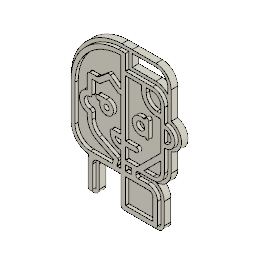
femIT_keychain (Autodesk Fusion 360 design; units mm, degrees)
Autodesk Fusion 360 part; units mm, degrees
sketch "MAIN" plane through (0, 0, 0) normal (0, 1, 0) x (1, 0, 0)
  line L0 (17.9916, -4.7059) -> (17.9916, -8.3513)
  line L1 (-9.0064, 3.7559) -> (-9.0064, -7.1582)
  line L2 (9.3752, 7.8431) -> (9.3752, 7.3129)
  arc A0 (12.3525, -3.3087) -> (13.2635, -3.4243) centre (12.8027, -3.4084) cw
  line L3 (3.167, 0.9058) -> (4.7357, 0.9058)
  line L4 (0.5265, -7.4454) -> (-1.9697, -7.4454)
  circle A1 centre (0.5265, -5.3563) radius 0.773
  arc A2 (-1.7946, -12.1762) -> (-2.4001, -11.97) centre (-2.4001, -12.9622) ccw
  arc A3 (18.0688, -9.5664) -> (17.9916, -9.6548) centre (18.0808, -9.6548) ccw
  spline S0 degree 3 poles (6.3043, 5.5675) (6.2676, 5.5675) (6.238, 5.5379) (6.238, 5.5012) knots 0 0 0 0 1 1 1 1
  spline S1 degree 3 poles (15.8928, 11.4887) (15.8928, 9.8013) (14.52, 8.4286) (12.8328, 8.4286) knots 0 0 0 0 1 1 1 1
  line L5 (6.3043, 6.7384) -> (7.8729, 6.7384)
  line L6 (4.5195, -12.2526) -> (1.6695, -14.3514)
  arc A4 (13.352, 9.8755) -> (14.4567, 11.0258) centre (13.352, 10.9811) ccw
  arc A5 (4.7303, -21.1201) -> (4.7964, -21.0671) centre (4.7314, -21.0537) ccw
  line L7 (4.7356, -12.2397) -> (4.5589, -12.2397)
  line L8 (2.5786, 7.2131) -> (2.2251, 8.3619)
  line L9 (-2.3821, 4.7038) -> (2.5445, 7.1341)
  arc A6 (12.1671, -8.257) -> (11.649, -8.0278) centre (11.8064, -8.3722) ccw
  arc A7 (-5.15, 9.5279) -> (-4.9416, 10.21) centre (-5.2035, 9.9172) ccw
  line L10 (6.238, -17.7188) -> (6.238, -22.2923)
  line L11 (7.9394, 6.8047) -> (7.9394, 8.3734)
  line L12 (9.6625, 5.5675) -> (6.3043, 5.5675)
  line L13 (-10.1773, -7.4786) -> (-10.1773, 3.865)
  line L14 (6.238, -22.2923) -> (4.1436, -22.2923)
  arc A8 (-5.2726, -7.0697) -> (-5.3234, -7.0131) centre (-5.3389, -7.0782) ccw
  arc A9 (-5.3234, -7.0131) -> (-5.3234, -1.1028) centre (-4.619, -4.058) cw
  arc A10 (4.7357, 2.1526) -> (3.1081, 0.9938) centre (4.7357, 0.4303) ccw
  arc A11 (-4.5662, -11.97) -> (-5.2726, -11.253) centre (-4.5556, -11.253) cw
  line L15 (17.9916, -9.6548) -> (17.9916, -14.0624)
  line L16 (4.7964, -21.0671) -> (4.8019, -12.306)
  arc A12 (-1.9697, -7.4454) -> (-1.9697, -6.0092) centre (-1.9697, -6.7273) cw
  arc A13 (18.0579, -4.6396) -> (17.9916, -4.7059) centre (18.0579, -4.7059) ccw
  line L17 (4.8019, 9.942) -> (4.8019, 17.8735)
  arc A14 (-5.2726, 0) -> (-2.3821, 4.7038) centre (0, 0) cw
  arc A15 (12.0111, -3.4605) -> (12.3525, -3.3087) centre (12.1257, -3.2584) ccw
  line L18 (-5.2726, -1.0382) -> (-5.2726, 0)
  arc A16 (9.4415, 0.5523) -> (9.4194, 1.9884) centre (9.4194, 1.2702) ccw
  arc A17 (13.2635, -8.0861) -> (12.1671, -8.257) centre (12.702, -8.0861) cw
  arc A18 (4.5589, -12.2397) -> (4.5195, -12.2526) centre (4.5587, -12.3059) ccw
  spline S2 degree 3 poles (6.3043, 17.4095) (6.2676, 17.4095) (6.238, 17.3799) (6.238, 17.3432) knots 0 0 0 0 1 1 1 1
  arc A19 (6.3043, -17.6525) -> (6.238, -17.7188) centre (6.3043, -17.7188) ccw
  line L19 (6.3043, 9.8755) -> (13.352, 9.8755)
  arc A20 (2.2251, 8.3619) -> (2.1616, 8.4085) centre (2.162, 8.3425) ccw
  arc A21 (17.9916, -8.3513) -> (18.0579, -8.4175) centre (18.0579, -8.3513) ccw
  spline S3 degree 3 poles (-10.1773, 3.865) (-10.1256, 6.7548) (-8.012, 9.1345) (-5.15, 9.5279) knots 0 0 0 0 1 1 1 1
  arc A22 (11.649, -8.0278) -> (12.0111, -3.4605) centre (10.7656, -5.6598) cw
  arc A23 (6.238, 2.0547) -> (6.3043, 1.9884) centre (6.3043, 2.0547) ccw
  line L20 (-5.2726, -11.253) -> (-5.2726, -7.0697)
  spline S4 degree 3 poles (9.9607, 8.4286) (9.6378, 8.4286) (9.3752, 8.1661) (9.3752, 7.8431) knots 0 0 0 0 1 1 1 1
  line L21 (0.7791, -14.3317) -> (-1.7946, -12.1762)
  line L22 (15.6827, -10.4943) -> (16.7544, -10.4943)
  arc A24 (-4.3557, 8.4085) -> (-9.0064, 3.7559) centre (-4.3557, 3.7579) ccw
  line L23 (5.7851, 18.8566) -> (14.9096, 18.8566)
  arc A25 (-1.5388, -6.0092) -> (-1.4815, -5.9331) centre (-1.5388, -5.9495) ccw
  arc A26 (-5.3234, -1.1028) -> (-5.2726, -1.0382) centre (-5.3388, -1.0385) ccw
  line L24 (6.238, 17.3432) -> (6.238, 9.942)
  line L25 (-1.9697, -6.0092) -> (-1.5388, -6.0092)
  line L26 (-2.4001, -11.97) -> (-4.5662, -11.97)
  arc A27 (-9.0064, -7.1582) -> (4.7303, -21.1201) centre (4.9573, -7.1582) ccw
  arc A28 (2.5445, 7.1341) -> (2.5786, 7.2131) centre (2.5152, 7.1936) ccw
  line L27 (2.1616, 8.4085) -> (-4.3557, 8.4085)
  circle A29 centre (4.7357, 2.0863) radius 0.0663
  spline S5 degree 3 poles (9.7092, 5.5482) (9.6969, 5.5605) (9.6799, 5.5675) (9.6625, 5.5675) knots 0 0 0 0 1 1 1 1
  line L28 (15.8928, 17.8735) -> (15.8928, 11.4887)
  arc A30 (1.6695, -14.3514) -> (0.7791, -14.3317) centre (1.2366, -13.7855) cw
  arc A31 (18.0579, -8.4175) -> (18.0579, -4.6396) centre (18.0579, -6.5286) ccw
  arc A32 (4.8019, -12.306) -> (4.7356, -12.2397) centre (4.7356, -12.306) ccw
  line L29 (6.238, 8.3734) -> (6.238, 6.8047)
  arc A33 (-1.4815, -5.9331) -> (0.5265, -7.4454) centre (0.5265, -5.3563) cw
  line L30 (13.2635, -3.4243) -> (13.2635, -8.0861)
  spline S6 degree 3 poles (-3.8353, 0.0055) (-3.8354, 0.0037) (-3.8365, 0.002) (-3.8365, 0) knots 0 0 0 0 1 1 1 1
  spline S7 degree 3 poles (7.9394, 8.3734) (7.9394, 8.41) (7.9095, 8.4396) (7.8729, 8.4396) knots 0 0 0 0 1 1 1 1
  line L31 (16.8209, 0.6188) -> (16.8209, 3.4024)
  spline S8 degree 3 poles (7.8729, 6.7384) (7.9095, 6.7384) (7.9394, 6.7681) (7.9394, 6.8047) knots 0 0 0 0 1 1 1 1
  arc A34 (3.1081, 0.9938) -> (3.1707, 0.9058) centre (3.1707, 0.9721) ccw
  line L32 (7.8729, 8.4396) -> (6.3043, 8.4396)
  spline S9 degree 3 poles (14.9096, 18.8566) (15.4516, 18.8566) (15.8928, 18.4155) (15.8928, 17.8735) knots 0 0 0 0 1 1 1 1
  line L33 (4.8019, 3.7021) -> (4.8019, 8.3513)
  arc A35 (14.3904, -17.6525) -> (17.9916, -14.0624) centre (14.3904, -14.0513) ccw
  spline S10 degree 3 poles (4.7357, 9.8755) (4.7723, 9.8755) (4.8019, 9.9052) (4.8019, 9.942) knots 0 0 0 0 1 1 1 1
  spline S11 degree 3 poles (6.238, 9.942) (6.238, 9.9052) (6.2676, 9.8755) (6.3043, 9.8755) knots 0 0 0 0 1 1 1 1
  arc A36 (4.7357, 0.9058) -> (4.8019, 0.9721) centre (4.7357, 0.9721) ccw
  arc A37 (16.7544, -10.4943) -> (16.8209, -10.428) centre (16.7544, -10.4278) ccw
  line L34 (14.6553, 5.5675) -> (11.8716, 5.5675)
  line L35 (-2.047, 9.8755) -> (4.7357, 9.8755)
  arc A38 (17.9916, 3.1373) -> (14.3794, 6.7274) centre (14.3794, 3.1151) ccw
  arc A39 (16.7074, 0.5718) -> (16.8209, 0.6188) centre (16.7544, 0.6188) ccw
  arc A40 (-3.6596, 11.4887) -> (-2.047, 9.8755) centre (-2.0464, 11.4887) ccw
  line L36 (11.8248, 5.4543) -> (16.7074, 0.5718)
  arc A41 (5.7851, 18.8566) -> (4.8019, 17.8735) centre (5.7851, 17.8735) ccw
  arc A42 (-3.6596, 18.1167) -> (-5.0959, 18.1167) centre (-4.3777, 18.1167) ccw
  arc A43 (11.8716, 5.5675) -> (11.8248, 5.4543) centre (11.8717, 5.5012) ccw
  arc A44 (-10.1773, -7.4786) -> (4.1436, -22.2923) centre (4.6449, -7.4786) ccw
  spline S12 degree 3 poles (14.4567, 17.3432) (14.4567, 17.3799) (14.4271, 17.4095) (14.3904, 17.4095) knots 0 0 0 0 1 1 1 1
  spline S13 degree 3 poles (-3.8365, 0.011) (-3.8365, 0.0092) (-3.8354, 0.0074) (-3.8353, 0.0055) knots 0 0 0 0 1 1 1 1
  line L37 (4.7356, -0.5302) -> (2.206, -0.5302)
  spline S14 degree 3 poles (6.3043, 8.4396) (6.2676, 8.4396) (6.238, 8.41) (6.238, 8.3734) knots 0 0 0 0 1 1 1 1
  arc A45 (2.206, -0.5302) -> (1.5982, 0.0773) centre (2.206, 0.0775) cw
  line L38 (14.4567, 11.0258) -> (14.4567, 17.3432)
  line L39 (12.8328, 8.4286) -> (9.9607, 8.4286)
  arc A46 (15.6827, -10.4943) -> (11.0543, -15.1118) centre (15.6718, -15.1118) ccw
  arc A47 (-5.0959, 10.5483) -> (-4.9416, 10.21) centre (-4.633, 10.5551) ccw
  line L40 (14.3904, 17.4095) -> (6.3043, 17.4095)
  line L41 (1.5982, 0.0773) -> (1.5982, 0.4419)
  line L42 (4.8019, 0.9721) -> (4.8019, 2.0863)
  arc A48 (6.3043, 0.5523) -> (6.238, 0.4861) centre (6.3043, 0.4861) ccw
  arc A49 (4.6891, 3.5983) -> (4.8019, 3.7021) centre (4.6977, 3.7021) ccw
  arc A50 (10.9881, -16.4814) -> (11.0543, -16.4151) centre (10.9881, -16.4151) ccw
  arc A51 (1.5982, 0.4419) -> (4.6891, 3.5983) centre (4.7553, 0.4419) cw
  line L43 (-5.0959, 10.5483) -> (-5.0959, 18.1167)
  arc A52 (16.8209, 3.4024) -> (14.6553, 5.5675) centre (14.6553, 3.402) ccw
  arc A53 (4.8019, 8.3513) -> (4.7356, 8.4175) centre (4.7356, 8.3513) ccw
  arc A54 (18.0025, -3.3804) -> (18.0688, -3.4465) centre (18.0688, -3.3803) ccw
  line L44 (-3.6596, 18.1167) -> (-3.6596, 11.4887)
  arc A55 (18.0688, -9.5664) -> (18.0688, -3.4465) centre (18.0688, -6.5065) ccw
  line L45 (9.9607, 6.7274) -> (14.3794, 6.7274)
  circle A56 centre (10.7656, -5.6598) radius 1.2113
  spline S15 degree 3 poles (6.238, 6.8047) (6.238, 6.7681) (6.2676, 6.7384) (6.3043, 6.7384) knots 0 0 0 0 1 1 1 1
  line L46 (4.7356, 8.4175) -> (3.6974, 8.4175)
  arc A57 (6.238, -16.4151) -> (6.3043, -16.4814) centre (6.3043, -16.4151) ccw
  arc A58 (-1.6686, 3.4447) -> (-3.8365, 0) centre (-0.0158, 0) ccw
  arc A59 (4.1181, 6.7692) -> (3.8886, 6.2231) centre (3.6781, 6.6329) cw
  line L47 (-3.8365, 0) -> (-3.8365, -1.705)
  line L48 (3.6341, 8.3317) -> (4.1181, 6.7692)
  line L49 (3.8886, 6.2231) -> (-1.6686, 3.4447)
  arc A60 (3.6974, 8.4175) -> (3.6341, 8.3317) centre (3.6974, 8.3513) ccw
  arc A61 (-4.5807, -5.6331) -> (-3.8365, -6.3629) centre (-4.5607, -6.357) cw
  line L50 (6.3043, -16.4814) -> (10.9881, -16.4814)
  line L51 (-3.7703, -10.5385) -> (-1.5188, -10.5385)
  arc A62 (16.8209, -11.9967) -> (16.7544, -11.9304) centre (16.7544, -11.9968) ccw
  arc A63 (14.3904, -16.4814) -> (16.8209, -14.0734) centre (14.3904, -14.0509) ccw
  line L52 (17.9916, 3.1373) -> (18.0025, -3.3804)
  line L53 (16.8013, -1.5438) -> (9.7092, 5.5482)
  arc A64 (-4.6209, -2.4303) -> (-4.5807, -5.6331) centre (-4.6209, -4.0319) ccw
  arc A65 (1.2243, -12.8428) -> (1.3064, -12.8454) centre (1.267, -12.792) ccw
  line L54 (11.0543, -16.4151) -> (11.0543, -15.1118)
  line L55 (16.8209, -14.0734) -> (16.8209, -11.9967)
  arc A66 (-3.8365, -1.705) -> (-4.6209, -2.4303) centre (-4.6209, -1.6435) cw
  line L56 (12.5567, -16.4814) -> (14.3904, -16.4814)
  line L57 (-3.8365, -6.3629) -> (-3.8365, -10.4722)
  arc A67 (4.8019, -0.5965) -> (4.7356, -0.5302) centre (4.7356, -0.5965) ccw
  line L58 (6.238, 0.4861) -> (6.238, -16.4151)
  line L59 (4.0725, -10.8036) -> (4.7356, -10.8036)
  arc A68 (4.7356, -10.8036) -> (4.8019, -10.7373) centre (4.7356, -10.7373) ccw
  line L60 (1.3064, -12.8454) -> (4.0725, -10.8036)
  arc A69 (-3.8365, -10.4722) -> (-3.7703, -10.5385) centre (-3.7703, -10.4722) ccw
  line L61 (4.8019, -10.7373) -> (4.8019, -0.5965)
  line L62 (-1.5188, -10.5385) -> (1.2243, -12.8428)
  line L63 (9.4415, 0.5523) -> (6.3043, 0.5523)
  arc A70 (12.4904, -16.4151) -> (12.5567, -16.4814) centre (12.5567, -16.4151) ccw
  spline S16 degree 3 poles (9.3752, 7.3129) (9.3752, 6.9901) (9.6378, 6.7274) (9.9607, 6.7274) knots 0 0 0 0 1 1 1 1
  line L64 (12.4904, -15.1118) -> (12.4904, -16.4151)
  line L65 (6.238, 5.5012) -> (6.238, 2.0547)
  line L66 (6.3043, 1.9884) -> (9.4194, 1.9884)
  line L67 (16.8209, -10.428) -> (16.8209, -1.5907)
  arc A71 (15.6718, -11.9304) -> (12.4904, -15.1118) centre (15.6718, -15.1118) ccw
  line L68 (16.7544, -11.9304) -> (15.6718, -11.9304)
  line L69 (14.3904, -17.6525) -> (6.3043, -17.6525)
  spline S17 degree 3 poles (16.8209, -1.5907) (16.8209, -1.573) (16.8137, -1.5563) (16.8013, -1.5438) knots 0 0 0 0 1 1 1 1
  line L70 (7.238, -23.2923) -> (4.1269, -23.2923)
  arc A72 (-11.1773, -7.4786) -> (4.1269, -23.2923) centre (4.6449, -7.4786) ccw
  line L71 (-11.1773, -7.4786) -> (-11.1773, 3.874)
  spline S18 degree 3 poles (-11.1773, 3.874) (-11.1773, 3.877) (-11.1772, 3.88) (-11.1772, 3.8829) (-11.1218, 6.9765) (-9.0162, 9.6026) (-6.083, 10.3615) knots -0.001032 -0.001032 -0.001032 -0.001032 0 0 0 0.918689 0.918689 0.918689 0.918689
  arc A73 (-6.0959, 10.5429) -> (-6.083, 10.3615) centre (-4.633, 10.5551) ccw
  line L72 (-6.0959, 10.5429) -> (-6.0959, 18.1167)
  arc A74 (-2.6596, 18.1167) -> (-6.0959, 18.1167) centre (-4.3777, 18.1167) ccw
  line L73 (-2.6596, 18.1167) -> (-2.6596, 11.4887)
  arc A75 (-2.6596, 11.4887) -> (-2.0462, 10.8755) centre (-2.0464, 11.4887) ccw
  line L74 (-2.0462, 10.8755) -> (3.8019, 10.8755)
  line L75 (3.8019, 10.8755) -> (3.8019, 17.8735)
  arc A76 (5.7851, 19.8566) -> (3.8019, 17.8735) centre (5.7851, 17.8735) ccw
  line L76 (5.7851, 19.8566) -> (14.9096, 19.8566)
  spline S19 degree 3 poles (14.9096, 19.8566) (15.8842, 19.8566) (16.7097, 19.1405) (16.866, 18.1986) (16.8837, 18.0923) (16.8928, 17.9834) (16.8928, 17.8735) knots 0 0 0 0 0.898599 0.898599 0.898599 1 1 1 1
  line L77 (16.8928, 17.8735) -> (16.8928, 11.4887)
  spline S20 degree 3 poles (16.8928, 11.4887) (16.8928, 9.7969) (15.8471, 8.3329) (14.3617, 7.7274) knots 0 0 0 0 0.758742 0.758742 0.758742 0.758742
  line L78 (14.3617, 7.7274) -> (14.3794, 7.7274)
  arc A77 (18.9916, 3.141) -> (14.3794, 7.7274) centre (14.3794, 3.1151) ccw
  line L79 (18.9916, 3.141) -> (19.0011, -2.5551)
  arc A78 (18.9916, -10.4601) -> (19.0011, -2.5551) centre (18.0688, -6.5065) ccw
  line L80 (18.9916, -10.4601) -> (18.9916, -14.0638)
  arc A79 (14.3904, -18.6525) -> (18.9916, -14.0638) centre (14.3904, -14.0513) ccw
  line L81 (14.3904, -18.6525) -> (7.238, -18.6525)
  line L82 (7.238, -18.6525) -> (7.238, -23.2923)
  line L83 (7.238, -23.2923) -> (21.9939, -23.2923)
  line L84 (18.9916, -14.0638) -> (18.9916, -25.254)
  arc A80 (14.3904, -23.2923) -> (18.9916, -18.6911) centre (14.3904, -18.6911) ccw
  arc A81 (14.3904, -22.2923) -> (17.9916, -18.6911) centre (14.3904, -18.6911) ccw
  line L85 (14.3904, -22.2923) -> (7.238, -22.2923)
  line L86 (17.9916, -18.6911) -> (17.9916, -16.9153)
  line L87 (5.7851, 19.8566) -> (-4.3777, 19.8348)
  dimension "d6" = 1
  dimension "d7" = -1
  constraint horizontal L83
  constraint perpendicular L82 L83
  constraint vertical L84
  constraint tangent L83 A80
  constraint tangent L84 A80
  constraint equal A79 A80
  constraint coincident L83 A80.start
  constraint coincident L84 A80.end
  constraint coincident L82 L85.end
  constraint tangent A81 L85
  constraint perpendicular L82 L85
  constraint coincident A79 L86.end
  constraint tangent A81 L86
  constraint vertical L86
  constraint midpoint A74 L87.end
extrude "Extrude1" add sketch "MAIN" along normal blind 2 contours L0 A13 A21 A31 | L1 A2 L6 A5 L7 L8 L9 A8 A9 A11 L16 A14 L18 A18 A20 L20 L21 A24 A26 L26 A27 A28 L27 A30 A32 | L2 A3 S1 A7 L10 L13 L14 L15 L17 A19 S3 S4 L23 L28 S9 A35 S10 L35 A38 A40 A41 A42 A44 L39 A47 L43 A54 L44 A55 L45 L52 S16 L69 | A0 A6 A15 A17 A22 L30 | L3 A10 A29 A34 A36 L42 | L4 A12 A25 L25 A33 | A1 | S0 L12 A16 A23 L22 S5 A37 A46 A48 A50 A57 L50 L53 L54 L58 L63 L65 L66 L67 S17 | L5 L11 L29 S7 S8 L32 S14 S15 | A4 S2 L19 L24 S11 S12 L38 L40 | L33 L37 A45 L41 A49 A51 A53 L46 A58 A59 L47 L48 L49 A60 A61 L51 A64 A65 A66 L57 A67 L59 A68 L60 A69 L61 L62 | L31 L34 A39 L36 A43 A52 | A56 | A62 A63 L55 L56 A70 L64 A71 L68 | L70 A72 L71 S18 A73 L72 A74 L73 A75 L74 L75 A76 L76 S19 L77 S20 A77 L79 A78 L80 A79 L81 L82 | A79 L82 L83 L84 A80 A81 L85 L86
extrude "Extrude2" add sketch "MAIN" against normal blind 1 contours L2 A3 S1 A7 L10 L13 L14 L15 L17 A19 S3 S4 L23 L28 S9 A35 S10 L35 A38 A40 A41 A42 A44 L39 A47 L43 A54 L44 A55 L45 L52 S16 L69 | A0 A6 A15 A17 A22 L30 | L4 A12 A25 L25 A33
